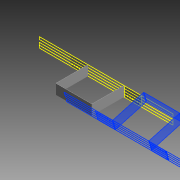
# Autodesk Inventor part: battery staple
Saved by Autodesk Inventor 2014 SP1 (Build 180222100, 222)
## iProperties
Created: 2014-01-07
Part Number: battery staple
Material: Generic
Document SubType Name: Sheet Metal
Designer: Arpan
Density: 1 g/cm^3
Sheet Metal Rule: Default
Appearance: Default
Mass: 55.2856 g
Surface Area: 725.823 cm^2
Volume: 55.2856 cm^3
Author: Arpan
Autodesk Inventor part; units mm, degrees
ref_plane "YZ Plane" through (0, 0, 0) normal (1, 0, 0) x (0, 1, 0)
ref_plane "XZ Plane" through (0, 0, 0) normal (0, 1, 0) x (-1, 0, 0)
ref_plane "XY Plane" through (0, 0, 0) normal (0, 0, 1) x (1, 0, 0)
sketch "Sketch1" plane through (0, 0, 0) normal (0, 0, 1) x (1, 0, 0)
  line L0 (0, 0) -> (-184.15, 0)
  line L1 (-184.15, 0) -> (-184.15, 50.8)
  line L2 (-184.15, 50.8) -> (0, 50.8)
  line L3 (0, 50.8) -> (0, 0)
  dimension "d0" = 184.15
  dimension "d1" = 50.8
  measures "d0" distance of L1.end L2.end
  measures "d1" distance of L2.end L0.start
extrude "Plate1" add sketch "Sketch1" along normal blind 1.5875
sketch "Sketch2" plane through (0, 0, 0) normal (1, 0, 0) x (0, 1, 0)
  line L0 (50.8, 0) -> (0, 0)
  line L1 (0, 0) -> (0, -165.1)
  line L2 (0, -165.1) -> (50.8, -165.1)
  line L3 (50.8, -165.1) -> (50.8, 0)
  constraints: 6 end point, 1 horizontal, 1 perpendicular, 1 vertical
edge flange "Flange1" height 165.1 angle 90 thickness 1.5875 bend radius 1.27 thickness toward (1, 0, 0) relief straight relief width 1.5875 relief depth 0.7937 corner gap 1.5875 corner form 0 edges at (0, 25.4, 0) (-184.15, 25.4, 0) wall of the first edge with corners at (0, 50.8, 0) (0, 0, 0) (0, 0, -165.1) (0, 50.8, -165.1)
bend "Bend1"
corner "Corner1"
sketch "Sketch3" plane through (1.5875, 50.8, -165.1) normal (0, 0, -1) x (-1, 0, 0)
  line L0 (0, -50.8) -> (0, 0)
  line L1 (0, 0) -> (-88.9, 0)
  line L2 (-88.9, 0) -> (-88.9, -50.8)
  line L3 (-88.9, -50.8) -> (0, -50.8)
  constraints: 6 end point, 1 horizontal, 1 perpendicular, 1 vertical
edge flange "Flange2" height 88.9 angle 90 thickness 1.5875 bend radius 1.27 thickness toward (0, 0, -1) relief straight relief width 1.5875 relief depth 0.7937 corner gap 1.5875 corner form 0 edges at (1.5875, 25.4, -165.1) (-185.7375, 25.4, -165.1) wall of the first edge with corners at (1.5875, 0, -165.1) (1.5875, 50.8, -165.1) (90.4875, 50.8, -165.1) (90.4875, 0, -165.1)
bend "Bend2"
corner "Corner2"
fillet "Corner Round1" radius 6.35 4 edges at (-274.6375, 50.8, -165.8938) (-274.6375, 0, -165.8938) (90.4875, 50.8, -165.8938) (90.4875, 0, -165.8938)
sketch "Sketch4" plane through (2.8575, 0, -165.1) normal (0, 0, 1) x (1, 0, 0)
  arc A0 (81.28, 0) -> (87.63, 6.35) centre (81.28, 6.35) ccw projected
  line L0 (87.63, 6.35) -> (87.63, 44.45) projected
  arc A1 (87.63, 44.45) -> (81.28, 50.8) centre (81.28, 44.45) ccw projected
  line L1 (81.28, 50.8) -> (0, 50.8) projected
  line L2 (0, 50.8) -> (0, 0) projected
  line L3 (81.28, 0) -> (0, 0) projected
  point P0 (-2.8575, 0)
sketch "Sketch5" plane through (2.8575, 0, -165.1) normal (0, 0, 1) x (1, 0, 0)
  arc A0 (81.28, 0) -> (87.63, 6.35) centre (81.28, 6.35) ccw projected
  line L0 (249.555, 38.1762) -> (249.555, 50.8) projected
  line L1 (249.555, 50.8) -> (-439.42, 50.8) projected
  line L2 (-439.42, 50.8) -> (-439.42, 38.1762) projected
  line L3 (249.555, 38.1762) -> (-439.42, 38.1762) projected
  arc A1 (-216.9045, 12.7762) -> (-221.7535, 12.7762) centre (-219.329, 12.7) ccw projected
  line L4 (-209.0535, 12.7762) -> (-216.9045, 12.7762) projected
  arc A2 (-204.2045, 12.7762) -> (-209.0535, 12.7762) centre (-206.629, 12.7) ccw projected
  line L5 (13.8315, 12.7762) -> (-204.2045, 12.7762) projected
  arc A3 (18.6805, 12.7762) -> (13.8315, 12.7762) centre (16.256, 12.7) ccw projected
  line L6 (26.5315, 12.7762) -> (18.6805, 12.7762) projected
  arc A4 (31.3805, 12.7762) -> (26.5315, 12.7762) centre (28.956, 12.7) ccw projected
  line L7 (39.2315, 12.7762) -> (31.3805, 12.7762) projected
  arc A5 (44.0805, 12.7762) -> (39.2315, 12.7762) centre (41.656, 12.7) ccw projected
  line L8 (51.9315, 12.7762) -> (44.0805, 12.7762) projected
  arc A6 (56.7805, 12.7762) -> (51.9315, 12.7762) centre (54.356, 12.7) ccw projected
  line L9 (64.6315, 12.7762) -> (56.7805, 12.7762) projected
  arc A7 (69.4805, 12.7762) -> (64.6315, 12.7762) centre (67.056, 12.7) ccw projected
  line L10 (77.3315, 12.7762) -> (69.4805, 12.7762) projected
  arc A8 (82.1805, 12.7762) -> (77.3315, 12.7762) centre (79.756, 12.7) ccw projected
  line L11 (249.555, 12.7762) -> (82.1805, 12.7762) projected
  line L12 (249.555, 12.7762) -> (249.555, 25.3238) projected
  line L13 (249.555, 25.3238) -> (-439.42, 25.3238) projected
  line L14 (-439.42, 25.3238) -> (-439.42, 12.7762) projected
  line L15 (-272.5535, 12.7762) -> (-439.42, 12.7762) projected
  arc A9 (-267.7045, 12.7762) -> (-272.5535, 12.7762) centre (-270.129, 12.7) ccw projected
  line L16 (-259.8535, 12.7762) -> (-267.7045, 12.7762) projected
  arc A10 (-255.0045, 12.7762) -> (-259.8535, 12.7762) centre (-257.429, 12.7) ccw projected
  line L17 (-247.1535, 12.7762) -> (-255.0045, 12.7762) projected
  arc A11 (-242.3045, 12.7762) -> (-247.1535, 12.7762) centre (-244.729, 12.7) ccw projected
  line L18 (-234.4535, 12.7762) -> (-242.3045, 12.7762) projected
  arc A12 (-229.6045, 12.7762) -> (-234.4535, 12.7762) centre (-232.029, 12.7) ccw projected
  line L19 (-221.7535, 12.7762) -> (-229.6045, 12.7762) projected
  arc A13 (-221.7535, 12.6238) -> (-216.9045, 12.6238) centre (-219.329, 12.7) ccw projected
  line L20 (-221.7535, 12.6238) -> (-229.6045, 12.6238) projected
  arc A14 (-234.4535, 12.6238) -> (-229.6045, 12.6238) centre (-232.029, 12.7) ccw projected
  line L21 (-234.4535, 12.6238) -> (-242.3045, 12.6238) projected
  arc A15 (-247.1535, 12.6238) -> (-242.3045, 12.6238) centre (-244.729, 12.7) ccw projected
  line L22 (-247.1535, 12.6238) -> (-255.0045, 12.6238) projected
  arc A16 (-259.8535, 12.6238) -> (-255.0045, 12.6238) centre (-257.429, 12.7) ccw projected
  line L23 (-259.8535, 12.6238) -> (-267.7045, 12.6238) projected
  arc A17 (-272.5535, 12.6238) -> (-267.7045, 12.6238) centre (-270.129, 12.7) ccw projected
  line L24 (-272.5535, 12.6238) -> (-439.42, 12.6238) projected
  line L25 (-439.42, 12.6238) -> (-439.42, 0) projected
  line L26 (249.555, 0) -> (-439.42, 0) projected
  line L27 (249.555, 0) -> (249.555, 12.6238) projected
  line L28 (249.555, 12.6238) -> (82.1805, 12.6238) projected
  arc A18 (77.3315, 12.6238) -> (82.1805, 12.6238) centre (79.756, 12.7) ccw projected
  line L29 (77.3315, 12.6238) -> (69.4805, 12.6238) projected
  arc A19 (64.6315, 12.6238) -> (69.4805, 12.6238) centre (67.056, 12.7) ccw projected
  line L30 (64.6315, 12.6238) -> (56.7805, 12.6238) projected
  arc A20 (51.9315, 12.6238) -> (56.7805, 12.6238) centre (54.356, 12.7) ccw projected
  line L31 (51.9315, 12.6238) -> (44.0805, 12.6238) projected
  arc A21 (39.2315, 12.6238) -> (44.0805, 12.6238) centre (41.656, 12.7) ccw projected
  line L32 (39.2315, 12.6238) -> (31.3805, 12.6238) projected
  arc A22 (26.5315, 12.6238) -> (31.3805, 12.6238) centre (28.956, 12.7) ccw projected
  line L33 (26.5315, 12.6238) -> (18.6805, 12.6238) projected
  arc A23 (13.8315, 12.6238) -> (18.6805, 12.6238) centre (16.256, 12.7) ccw projected
  line L34 (13.8315, 12.6238) -> (-204.2045, 12.6238) projected
  arc A24 (-209.0535, 12.6238) -> (-204.2045, 12.6238) centre (-206.629, 12.7) ccw projected
  line L35 (-209.0535, 12.6238) -> (-216.9045, 12.6238) projected
  circle A25 centre (-270.129, 12.7) radius 2.4257
  circle A26 centre (-244.729, 12.7) radius 2.4257
  circle A27 centre (-257.429, 12.7) radius 2.4257
  circle A28 centre (-232.029, 12.7) radius 2.4257
  circle A29 centre (-219.329, 12.7) radius 2.4257
  circle A30 centre (-206.629, 12.7) radius 2.4257
  circle A31 centre (16.256, 12.7) radius 2.4257
  circle A32 centre (28.956, 12.7) radius 2.4257
  circle A33 centre (41.656, 12.7) radius 2.4257
  circle A34 centre (54.356, 12.7) radius 2.4257
  circle A35 centre (67.056, 12.7) radius 2.4257
  circle A36 centre (79.756, 12.7) radius 2.4257
  arc A37 (-221.7535, 37.8714) -> (-216.9045, 37.8714) centre (-219.329, 37.9476) ccw
  line L36 (-209.0535, 37.8714) -> (-216.9045, 37.8714)
  arc A38 (-209.0535, 37.8714) -> (-204.2045, 37.8714) centre (-206.629, 37.9476) ccw
  line L37 (13.8315, 37.8714) -> (-204.2045, 37.8714)
  arc A39 (13.8315, 37.8714) -> (18.6805, 37.8714) centre (16.256, 37.9476) ccw
  line L38 (26.5315, 37.8714) -> (18.6805, 37.8714)
  arc A40 (26.5315, 37.8714) -> (31.3805, 37.8714) centre (28.956, 37.9476) ccw
  line L39 (39.2315, 37.8714) -> (31.3805, 37.8714)
  arc A41 (39.2315, 37.8714) -> (44.0805, 37.8714) centre (41.656, 37.9476) ccw
  line L40 (51.9315, 37.8714) -> (44.0805, 37.8714)
  arc A42 (51.9315, 37.8714) -> (56.7805, 37.8714) centre (54.356, 37.9476) ccw
  line L41 (64.6315, 37.8714) -> (56.7805, 37.8714)
  arc A43 (64.6315, 37.8714) -> (69.4805, 37.8714) centre (67.056, 37.9476) ccw
  line L42 (77.3315, 37.8714) -> (69.4805, 37.8714)
  arc A44 (77.3315, 37.8714) -> (82.1805, 37.8714) centre (79.756, 37.9476) ccw
  line L43 (249.555, 37.8714) -> (82.1805, 37.8714)
  arc A45 (-272.5535, 37.8714) -> (-267.7045, 37.8714) centre (-270.129, 37.9476) ccw
  line L44 (-259.8535, 37.8714) -> (-267.7045, 37.8714)
  arc A46 (-259.8535, 37.8714) -> (-255.0045, 37.8714) centre (-257.429, 37.9476) ccw
  line L45 (-247.1535, 37.8714) -> (-255.0045, 37.8714)
  arc A47 (-247.1535, 37.8714) -> (-242.3045, 37.8714) centre (-244.729, 37.9476) ccw
  line L46 (-234.4535, 37.8714) -> (-242.3045, 37.8714)
  arc A48 (-234.4535, 37.8714) -> (-229.6045, 37.8714) centre (-232.029, 37.9476) ccw
  line L47 (-221.7535, 37.8714) -> (-229.6045, 37.8714)
  arc A49 (-216.9045, 38.0238) -> (-221.7535, 38.0238) centre (-219.329, 37.9476) ccw
  line L48 (-221.7535, 38.0238) -> (-229.6045, 38.0238)
  arc A50 (-229.6045, 38.0238) -> (-234.4535, 38.0238) centre (-232.029, 37.9476) ccw
  line L49 (-234.4535, 38.0238) -> (-242.3045, 38.0238)
  arc A51 (-242.3045, 38.0238) -> (-247.1535, 38.0238) centre (-244.729, 37.9476) ccw
  line L50 (-247.1535, 38.0238) -> (-255.0045, 38.0238)
  arc A52 (-255.0045, 38.0238) -> (-259.8535, 38.0238) centre (-257.429, 37.9476) ccw
  line L51 (-259.8535, 38.0238) -> (-267.7045, 38.0238)
  arc A53 (-267.7045, 38.0238) -> (-272.5535, 38.0238) centre (-270.129, 37.9476) ccw
  line L52 (249.555, 38.0238) -> (82.1805, 38.0238)
  arc A54 (82.1805, 38.0238) -> (77.3315, 38.0238) centre (79.756, 37.9476) ccw
  line L53 (77.3315, 38.0238) -> (69.4805, 38.0238)
  arc A55 (69.4805, 38.0238) -> (64.6315, 38.0238) centre (67.056, 37.9476) ccw
  line L54 (64.6315, 38.0238) -> (56.7805, 38.0238)
  arc A56 (56.7805, 38.0238) -> (51.9315, 38.0238) centre (54.356, 37.9476) ccw
  line L55 (51.9315, 38.0238) -> (44.0805, 38.0238)
  arc A57 (44.0805, 38.0238) -> (39.2315, 38.0238) centre (41.656, 37.9476) ccw
  line L56 (39.2315, 38.0238) -> (31.3805, 38.0238)
  arc A58 (31.3805, 38.0238) -> (26.5315, 38.0238) centre (28.956, 37.9476) ccw
  line L57 (26.5315, 38.0238) -> (18.6805, 38.0238)
  arc A59 (18.6805, 38.0238) -> (13.8315, 38.0238) centre (16.256, 37.9476) ccw
  line L58 (13.8315, 38.0238) -> (-204.2045, 38.0238)
  arc A60 (-204.2045, 38.0238) -> (-209.0535, 38.0238) centre (-206.629, 37.9476) ccw
  line L59 (-209.0535, 38.0238) -> (-216.9045, 38.0238)
  circle A61 centre (-270.129, 37.9476) radius 2.4257
  circle A62 centre (-244.729, 37.9476) radius 2.4257
  circle A63 centre (-257.429, 37.9476) radius 2.4257
  circle A64 centre (-232.029, 37.9476) radius 2.4257
  circle A65 centre (-219.329, 37.9476) radius 2.4257
  circle A66 centre (-206.629, 37.9476) radius 2.4257
  circle A67 centre (16.256, 37.9476) radius 2.4257
  circle A68 centre (28.956, 37.9476) radius 2.4257
  circle A69 centre (41.656, 37.9476) radius 2.4257
  circle A70 centre (54.356, 37.9476) radius 2.4257
  circle A71 centre (67.056, 37.9476) radius 2.4257
  circle A72 centre (79.756, 37.9476) radius 2.4257
  point P0 (-2.8575, 0)
  point P1 (81.28, 44.2976)
  constraints: 87 symmetric about line, 24 coincident, 20 centre point, 8 concentric, 2 horizontal, 46 other
extrude "Cut1" cut sketch "Sketch5" against normal blind 1.5875 contours A54 A72 A44 L3 | L3 A54 | A55 A71 A43 L3 | L3 A55 | A53 L3 | L3 A53 A61 A45 | A56 A70 A42 L3 | L3 A56 | A52 L3 | L3 A52 A63 A46 | A57 A69 A41 L3 | L3 A57 | A51 L3 | L3 A51 A62 A47 | A58 A68 A40 L3 | L3 A58 | A50 L3 | L3 A50 A64 A48 | A59 A67 A39 L3 | L3 A59 | A49 L3 | L3 A49 A65 A37 | A60 A66 A38 L3 | L3 A60 | A29 A13 A1 | A2 A30 A24 | A28 A14 A12 | A3 A31 A23 | A26 A15 A11 | A4 A32 A22 | A27 A16 A10 | A5 A33 A21 | A25 A17 A9 | A6 A34 A20 | A7 A35 A19 | A8 A36 A18
equation "\"d24\" = Thickness"
equation "\"d3\" = BendReliefWidth"
equation "\"d4\" = BendReliefDepth"
equation "\"d5\" = MinimumRemnant"
equation "\"d6\" = BendRadius"
equation "\"d10\" = CornerReliefSize"
equation "\"d11\" = GapSize"
equation "\"d12\" = JacobiRadiusSize"
equation "\"d13\" = BendReliefWidth"
equation "\"d14\" = BendReliefDepth"
equation "\"d15\" = MinimumRemnant"
equation "\"d16\" = BendRadius"
equation "\"d20\" = CornerReliefSize"
equation "\"d21\" = GapSize"
equation "\"d22\" = JacobiRadiusSize"
equation "\"BendRadius\" = Thickness"
equation "\"BendReliefWidth\" = Thickness"
equation "\"BendReliefDepth\" = 0.5 * Thickness"
equation "\"CornerReliefSize\" = 4 * Thickness"
equation "\"MinimumRemnant\" = 2 * Thickness"
equation "\"TransitionRadius\" = BendRadius"
equation "\"JacobiRadiusSize\" = BendRadius"
equation "\"GapSize\" = Thickness"
equation "\"d2\" = BendRadius"
equation "\"Thickness\" = 1.5875"
body "Solid1"
